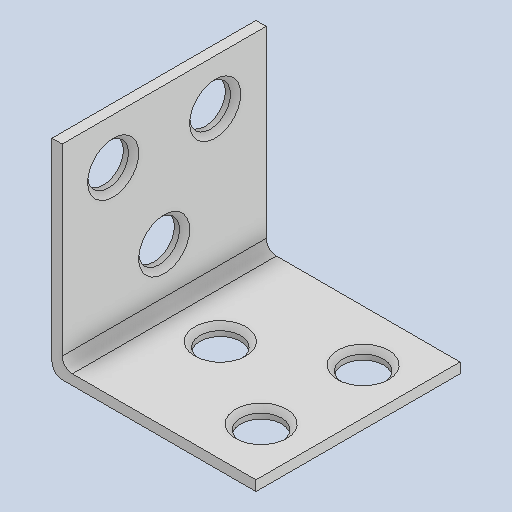
# Autodesk Inventor part: katownik_lacznikowy_40_40_40_CPY
Saved by Autodesk Inventor 2025.2 (Build 292293000, 293)
## iProperties
Created: 2025-03-19
Part Number: katownik_lacznikowy_40_40_40_CPY
Material: Ogólny
Document SubType Name: Modeling
Designer: tadek
Density: 1 g/cm^3
Appearance: Domyślna
Author: tadek
Autodesk Inventor part; units mm, degrees
ref_plane "YZ Plane" through (0, 0, 0) normal (1, 0, 0) x (0, 1, 0)
ref_plane "XZ Plane" through (0, 0, 0) normal (0, 1, 0) x (-1, 0, 0)
ref_plane "XY Plane" through (0, 0, 0) normal (0, 0, 1) x (1, 0, 0)
sketch "Szkic1" plane through (0, 0, 0) normal (0, 0, 1) x (1, 0, 0)
  line L0 (0, 2) -> (0, 40)
  line L1 (0, 40) -> (2, 40)
  line L2 (2, 40) -> (2, 4)
  line L3 (4, 2) -> (40, 2)
  line L4 (40, 2) -> (40, 0)
  line L5 (40, 0) -> (2, 0)
  arc A0 (0, 2) -> (2, 0) centre (2, 2) ccw
  arc A1 (2, 4) -> (4, 2) centre (4, 4) ccw
  point P0 (0, 0)
  point P1 (2, 2)
  dimension "d0" = 40
  dimension "d1" = 2
  dimension "d2" = 38
  dimension "d3" = 38
  dimension "d4" = 2
  constraints: 12 end point, 5 perpendicular, 4 point on circle, 4 point on line, 4 tangent, 2 centre point, 1 equal radius, 1 vertical
  measures "d0" distance of point (0, 0) L0.end
  measures "d1" distance of L0.end L1.end
  measures "d2" distance of L1.end point (2, 2)
  measures "d3" distance of point (2, 2) L3.end
  measures "d4" radius of A0
extrude "Wyciągnięcie proste1" add sketch "Szkic1" along normal blind 40
sketch "Szkic2" plane through (2, 4, 0) normal (1, 0, 0) x (0, 0, -1)
  line L0 (0, 0) -> (-40, 0) projected
  line L1 (-20, 0) -> (-20, 36)
  line L2 (0, 36) -> (-40, 36) projected
  line L3 (-20, 18) -> (-40, 18)
  line L4 (-40, 0) -> (-40, 36) projected
  line L5 (-20, 18) -> (0, 18)
  line L6 (-40, 18) -> (-40, 27)
  line L7 (-40, 27) -> (-30, 27)
  line L8 (0, 0) -> (0, 36) projected
  line L9 (0, 27) -> (-10, 27)
  line L10 (-20, 18) -> (-20, 9)
  point P0 (0, -4)
  dimension "d13" = 9
  dimension "d14" = 30
  dimension "d16" = 9
  dimension "d17" = 20
  dimension "d18" = 9
  constraints: 14 end point, 4 midpoint, 4 point on line, 2 perpendicular
  measures "d13" distance of L3.end L6.end
  measures "d14" distance from line of L8 L7.end
  measures "d16" distance between parallel lines of L5 L9
  measures "d17" diameter of L9.end L1
  measures "d18" distance of L3.start L10.end
sketch "Szkic3" plane through (4, 2, 0) normal (0, 1, 0) x (1, 0, 0)
  line L0 (0, 0) -> (0, -40) projected
  line L1 (0, -40) -> (0, -20)
  line L2 (0, -20) -> (9, -20)
  line L3 (36, -40) -> (0, -40) projected
  line L4 (18, -40) -> (18, 0)
  line L5 (36, 0) -> (0, 0) projected
  line L6 (18, -20) -> (36, -20)
  line L7 (36, 0) -> (36, -40) projected
  line L8 (27, -20) -> (27, -30)
  line L9 (27, -20) -> (27, -10)
  point P0 (-4, 0)
  dimension "d19" = 9
  dimension "d20" = 10
  dimension "d21" = 10
  constraints: 12 end point, 6 midpoint, 2 vertical, 1 horizontal
  measures "d19" distance of L1.end L2.end
  measures "d20" distance of L8.start L8.end
  measures "d21" distance of L8.start L9.end
hole "Otwór1" at (2, 31, 30) at (2, 31, 10) at (2, 13, 20) direction (-1, 0, 0) diameter 8 end through all countersink diameter 10 countersink angle 90
hole "Otwór2" at (13, 2, 20) at (31, 2, 30) at (31, 2, 10) direction (0, -1, 0) diameter 8 end through all countersink diameter 10 countersink angle 90
